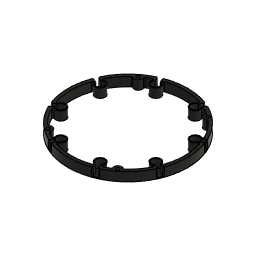
IR隠し (Autodesk Fusion 360 design; units mm, degrees)
Autodesk Fusion 360 part; units mm, degrees
sketch "スケッチ1" plane through (0, 0, 0) normal (0, 0, 1) x (1, 0, 0)
  circle A0 centre (0, 0) radius 60
  dimension "d1" = 120
  constraint coincident A0.centre origin
  measures "d1" diameter of A0
extrude "押し出し1" add sketch "スケッチ1" along normal blind 1.6 contours A0 picked at (15.326198, 22.479404)
sketch "スケッチ2" plane through (0, 0, 21.011891) normal (0, 0, 1) x (1, 0, 0)
  circle A0 centre (0, -1.188109) radius 1.5
  circle A1 centre (-35, -39.898109) radius 1.75
  circle A2 centre (35, -39.898109) radius 1.75
  circle A3 centre (-35, 45.311891) radius 1.75
  circle A4 centre (-35, -45.188109) radius 1.75
  circle A5 centre (35, 45.311891) radius 1.75
  circle A6 centre (35, -45.188109) radius 1.75
  line L0 (-40, 48.811891) -> (-40, -51.188109)
  line L1 (-40, -51.188109) -> (40, -51.188109)
  line L2 (40, -51.188109) -> (40, 48.811891)
  line L3 (40, 48.811891) -> (-40, 48.811891)
extrude "押し出し2" cut sketch "スケッチ2" against normal blind 45 contours A3 | A4 | A5 | A6 picked at (-35.557417, 45.483832) picked at (-35.557417, -45.016168) picked at (34.442583, 45.483832) picked at (34.442583, -45.016168)
sketch "スケッチ3" plane through (0, 0, 1.6) normal (0, 0, 1) x (-1, 0, 0)
  circle A0 centre (-35, 45.188109) radius 1.75
  circle A1 centre (-35, -45.311891) radius 1.75
  circle A2 centre (35, 45.188109) radius 1.75
  circle A3 centre (35, -45.311891) radius 1.75
  circle A4 centre (0, 0) radius 60
extrude "押し出し3" add sketch "スケッチ3" along normal blind 10 contours A4 picked at (11.241029, -14.670055)
extrude "押し出し4" cut 1 faces at (-11.241029, 14.670055, 11.6) along direction (0, 0, -1) blind 1.6
sketch "スケッチ4" plane through (0, 0, 10) normal (0, 0, 1) x (-1, 0, 0)
  circle A0 centre (-35, 45.188109) radius 1.75
  circle A1 centre (35, 45.188109) radius 1.75
  circle A2 centre (-35, -45.311891) radius 1.75
  circle A3 centre (35, -45.311891) radius 1.75
  circle A4 centre (0, 0) radius 60
  circle A5 centre (0, 0) radius 50
  dimension "d10" = 100
  constraint concentric A4 A5
  measures "d10" diameter of A5
extrude "押し出し5" cut sketch "スケッチ4" against normal blind 55 contours A5 picked at (-13.551782, -2.484038)
extrude "押し出し6" cut 1 faces at (-56.443283, 2.980845, 10) along direction (0, 0, -1) blind 1
sketch "スケッチ5" plane through (0, 0, 9) normal (0, 0, 1) x (-1, 0, 0)
  circle A0 centre (0, 0) radius 50
  circle A1 centre (-35, 45.188109) radius 1.75
  circle A2 centre (35, 45.188109) radius 1.75
  circle A3 centre (-35, -45.311891) radius 1.75
  circle A4 centre (35, -45.311891) radius 1.75
  circle A5 centre (0, 0) radius 60
  line L0 (0, 0) -> (0, 60)
  line L1 (0, 0) -> (22.961006, 55.432772)
  circle A6 centre (0, 0) radius 51.6
  circle A7 centre (19.746465, 47.672184) radius 4
  circle A8 centre (19.746465, 47.672184) radius 5
  circle A9 centre (-19.746465, 47.672184) radius 4
  circle A10 centre (-19.746465, 47.672184) radius 5
  circle A11 centre (-47.672184, 19.746465) radius 4
  circle A12 centre (-47.672184, 19.746465) radius 5
  circle A13 centre (-47.672184, -19.746465) radius 4
  circle A14 centre (-47.672184, -19.746465) radius 5
  circle A15 centre (-19.746465, -47.672184) radius 4
  circle A16 centre (-19.746465, -47.672184) radius 5
  circle A17 centre (19.746465, -47.672184) radius 4
  circle A18 centre (19.746465, -47.672184) radius 5
  circle A19 centre (47.672184, -19.746465) radius 4
  circle A20 centre (47.672184, -19.746465) radius 5
  circle A21 centre (47.672184, 19.746465) radius 4
  circle A22 centre (47.672184, 19.746465) radius 5
  dimension "d15" = 157.5
  dimension "d16" = 103.2
  dimension "d17" = 8
  dimension "d18" = 10
  dimension "d20" = 360
  constraint coincident A0.centre A5.centre
  constraint coincident A5 L0.end
  constraint vertical L0
  constraint concentric A7 A8
  measures "d15" angle of L0 L1
  measures "d16" diameter of A6
  measures "d17" diameter of A7
  measures "d18" diameter of A8
extrude "押し出し7" add sketch "スケッチ5" against normal blind 9 contours A0 A21 A22 | A0 A19 A20 | A0 L1 A7 A8 | A0 A17 A18 | A0 L1 A7 A8 | A0 A15 A16 | A0 A9 A10 | A0 A13 A14 | A0 A11 A12 picked at (43.248058, 18.291237) picked at (43.248058, -18.291237) picked at (22.313928, 43.786523) picked at (18.291237, -43.248058) picked at (15.183418, 46.740077) picked at (-22.308999, -43.783035) picked at (-22.308999, 43.783035) picked at (-46.768608, -15.177005) picked at (-46.768608, 15.177005)
extrude "押し出し8" cut sketch "スケッチ5" against normal blind 21 contours A0 A6 A21 | A0 A6 A19 | A6 A21 | A6 A19 | A0 L1 A6 A7 | A0 A6 A17 | A0 L1 A6 A7 | L1 A6 A7 | A6 A17 | L1 A6 A7 | A0 A6 A15 | A6 A15 | A0 A6 A9 | A6 A9 | A6 A13 | A0 A6 A13 | A0 A6 A11 | A6 A11 picked at (45.983245, 21.335973) picked at (45.983245, -21.335973) picked at (48.874047, 20.296753) picked at (48.874047, -20.296753) picked at (22.104519, 45.630587) picked at (17.428253, -47.601875) picked at (16.635442, 47.895953) picked at (21.000795, 48.527452) picked at (20.25766, -48.89118) picked at (19.466775, 49.163647) picked at (-21.335973, -45.983245) picked at (-20.252313, -48.893408) picked at (-21.335973, 45.983245) picked at (-20.252313, 48.893408) picked at (-48.893408, -20.252313) picked at (-47.601875, -17.428253) picked at (-47.601875, 17.428253) picked at (-48.893408, 20.252313)
sketch "スケッチ6" plane through (0, 0, 9) normal (0, 0, 1) x (-1, 0, 0)
  circle A0 centre (19.746465, -47.672184) radius 4
  circle A1 centre (19.746465, 47.672184) radius 4
  circle A2 centre (-47.672184, 19.746465) radius 4
  circle A3 centre (47.672184, -19.746465) radius 4
  circle A4 centre (-19.746465, -47.672184) radius 4
  circle A5 centre (-19.746465, 47.672184) radius 4
  circle A6 centre (-47.672184, -19.746465) radius 4
  circle A7 centre (47.672184, 19.746465) radius 4
  arc A8 (-23.354385, 44.21055) -> (-44.21055, 23.354385) centre (0, 0) ccw
  arc A9 (-23.354385, 44.21055) -> (-14.747535, 47.775624) centre (-19.746465, 47.672184) ccw
  arc A10 (14.747535, 47.775624) -> (-14.747535, 47.775624) centre (0, 0) ccw
  arc A11 (14.747535, 47.775624) -> (23.354385, 44.21055) centre (19.746465, 47.672184) ccw
  arc A12 (44.21055, 23.354385) -> (23.354385, 44.21055) centre (0, 0) ccw
  arc A13 (44.21055, 23.354385) -> (47.775624, 14.747535) centre (47.672184, 19.746465) ccw
  arc A14 (47.775624, -14.747535) -> (47.775624, 14.747535) centre (0, 0) ccw
  arc A15 (47.775624, -14.747535) -> (44.21055, -23.354385) centre (47.672184, -19.746465) ccw
  arc A16 (23.354385, -44.21055) -> (44.21055, -23.354385) centre (0, 0) ccw
  arc A17 (23.354385, -44.21055) -> (14.747535, -47.775624) centre (19.746465, -47.672184) ccw
  arc A18 (-14.747535, -47.775624) -> (14.747535, -47.775624) centre (0, 0) ccw
  arc A19 (-14.747535, -47.775624) -> (-23.354385, -44.21055) centre (-19.746465, -47.672184) ccw
  arc A20 (-44.21055, -23.354385) -> (-23.354385, -44.21055) centre (0, 0) ccw
  arc A21 (-44.21055, -23.354385) -> (-47.775624, -14.747535) centre (-47.672184, -19.746465) ccw
  arc A22 (-47.775624, 14.747535) -> (-47.775624, -14.747535) centre (0, 0) ccw
  arc A23 (-47.775624, 14.747535) -> (-44.21055, 23.354385) centre (-47.672184, 19.746465) ccw
  circle A24 centre (-35, 45.188109) radius 1.75
  circle A25 centre (35, 45.188109) radius 1.75
  circle A26 centre (-35, -45.311891) radius 1.75
  circle A27 centre (35, -45.311891) radius 1.75
  circle A28 centre (0, 0) radius 60
  line L0 (0, 0) -> (19.746465, 47.672184)
  line L1 (19.746465, 47.672184) -> (30.643995, 73.981148)
  line L2 (22.961006, 55.432772) -> (21.277199, 51.367702)
  line L3 (22.119102, 53.400237) -> (23.966861, 52.63487)
  line L4 (22.119102, 53.400237) -> (20.271343, 54.165604)
  line L5 (20.271343, 54.165604) -> (21.100487, 56.167334)
  line L6 (23.966861, 52.63487) -> (24.796005, 54.636601)
  line L7 (23.966861, 52.63487) -> (22.919878, 50.10723)
  line L8 (20.271343, 54.165604) -> (19.22436, 51.637963)
  line L9 (-23.966861, 52.63487) -> (-24.796005, 54.636601)
  line L10 (-23.966861, 52.63487) -> (-22.919878, 50.10723)
  line L11 (-20.271343, 54.165604) -> (-21.100487, 56.167334)
  line L12 (-20.271343, 54.165604) -> (-19.22436, 51.637963)
  line L13 (-54.165604, 20.271343) -> (-56.167334, 21.100487)
  line L14 (-54.165604, 20.271343) -> (-51.637963, 19.22436)
  line L15 (-52.63487, 23.966861) -> (-54.636601, 24.796005)
  line L16 (-52.63487, 23.966861) -> (-50.10723, 22.919878)
  line L17 (-52.63487, -23.966861) -> (-54.636601, -24.796005)
  line L18 (-52.63487, -23.966861) -> (-50.10723, -22.919878)
  line L19 (-54.165604, -20.271343) -> (-56.167334, -21.100487)
  line L20 (-54.165604, -20.271343) -> (-51.637963, -19.22436)
  line L21 (-20.271343, -54.165604) -> (-21.100487, -56.167334)
  line L22 (-20.271343, -54.165604) -> (-19.22436, -51.637963)
  line L23 (-23.966861, -52.63487) -> (-24.796005, -54.636601)
  line L24 (-23.966861, -52.63487) -> (-22.919878, -50.10723)
  line L25 (23.966861, -52.63487) -> (24.796005, -54.636601)
  line L26 (23.966861, -52.63487) -> (22.919878, -50.10723)
  line L27 (20.271343, -54.165604) -> (21.100487, -56.167334)
  line L28 (20.271343, -54.165604) -> (19.22436, -51.637963)
  line L29 (54.165604, -20.271343) -> (56.167334, -21.100487)
  line L30 (54.165604, -20.271343) -> (51.637963, -19.22436)
  line L31 (52.63487, -23.966861) -> (54.636601, -24.796005)
  line L32 (52.63487, -23.966861) -> (50.10723, -22.919878)
  line L33 (52.63487, 23.966861) -> (54.636601, 24.796005)
  line L34 (52.63487, 23.966861) -> (50.10723, 22.919878)
  line L35 (54.165604, 20.271343) -> (56.167334, 21.100487)
  line L36 (54.165604, 20.271343) -> (51.637963, 19.22436)
  dimension "d25" = 2
  dimension "d26" = 2
  dimension "d28" = 360
  constraint coincident A8.centre A10.centre
  constraint parallel L0 L1
  constraint perpendicular L1 L3
  constraint perpendicular L1 L4
  constraint perpendicular L4 L5
  constraint perpendicular L3 L6
  constraint perpendicular L3 L7
  constraint perpendicular L4 L8
extrude "押し出し9" cut sketch "スケッチ6" against normal blind 8 contours A0 A28 L25 L26 L27 L28 | A4 A28 L21 L22 L23 L24 | A3 A28 L29 L30 L31 L32 | A6 A28 L17 L18 L19 L20 | A7 A28 L33 L34 L35 L36 | A2 A28 L13 L14 L15 L16 | A28 L1 L2 L3 L6 | A5 A28 L9 L10 L11 L12 | A28 L1 L2 L4 L5 | A1 L1 L2 L3 L7 | A1 L1 L2 L4 L8 picked at (21.744986, -52.757411) picked at (-21.744986, -52.757411) picked at (52.722725, -21.838468) picked at (-52.68115, -21.929097) picked at (52.722725, 21.838468) picked at (-52.757411, 21.744986) picked at (23.424422, 53.647963) picked at (-21.929097, 52.68115) picked at (21.371271, 54.498406) picked at (22.61081, 52.390464) picked at (21.057396, 53.033909)
sketch "スケッチ7" plane through (0, 0, 0) normal (0, 0, -1) x (1, 0, 0)
  circle A0 centre (47.672184, 19.746465) radius 4
  circle A1 centre (-47.672184, -19.746465) radius 4
  circle A2 centre (19.746465, 47.672184) radius 4
  circle A3 centre (-19.746465, -47.672184) radius 4
  circle A4 centre (47.672184, -19.746465) radius 4
  circle A5 centre (-47.672184, 19.746465) radius 4
  circle A6 centre (-19.746465, 47.672184) radius 4
  circle A7 centre (19.746465, -47.672184) radius 4
  arc A8 (44.21055, 23.354385) -> (47.775624, 14.747535) centre (47.672184, 19.746465) ccw
  arc A9 (47.775624, -14.747535) -> (47.775624, 14.747535) centre (0, 0) ccw
  arc A10 (47.775624, -14.747535) -> (44.21055, -23.354385) centre (47.672184, -19.746465) ccw
  arc A11 (23.354385, -44.21055) -> (44.21055, -23.354385) centre (0, 0) ccw
  arc A12 (23.354385, -44.21055) -> (14.747535, -47.775624) centre (19.746465, -47.672184) ccw
  arc A13 (-14.747535, -47.775624) -> (14.747535, -47.775624) centre (0, 0) ccw
  arc A14 (-14.747535, -47.775624) -> (-23.354385, -44.21055) centre (-19.746465, -47.672184) ccw
  arc A15 (-44.21055, -23.354385) -> (-23.354385, -44.21055) centre (0, 0) ccw
  arc A16 (-44.21055, -23.354385) -> (-47.775624, -14.747535) centre (-47.672184, -19.746465) ccw
  arc A17 (-47.775624, 14.747535) -> (-47.775624, -14.747535) centre (0, 0) ccw
  arc A18 (-47.775624, 14.747535) -> (-44.21055, 23.354385) centre (-47.672184, 19.746465) ccw
  arc A19 (-23.354385, 44.21055) -> (-44.21055, 23.354385) centre (0, 0) ccw
  arc A20 (-23.354385, 44.21055) -> (-14.747535, 47.775624) centre (-19.746465, 47.672184) ccw
  arc A21 (14.747535, 47.775624) -> (-14.747535, 47.775624) centre (0, 0) ccw
  arc A22 (14.747535, 47.775624) -> (23.354385, 44.21055) centre (19.746465, 47.672184) ccw
  arc A23 (44.21055, 23.354385) -> (23.354385, 44.21055) centre (0, 0) ccw
  circle A24 centre (35, 45.188109) radius 1.75
  circle A25 centre (35, -45.311891) radius 1.75
  circle A26 centre (-35, 45.188109) radius 1.75
  circle A27 centre (-35, -45.311891) radius 1.75
  circle A28 centre (0, 0) radius 60
extrude "押し出し10" add sketch "スケッチ7" against normal blind 1 contours A0 | A1 | A2 | A3 | A4 | A5 | A6 | A7 picked at (48.338851, 21.687179) picked at (-48.901937, -19.945188) picked at (18.600469, 46.726807) picked at (-18.915145, -49.112072) picked at (46.442431, -19.945188) picked at (-47.005517, 21.687179) picked at (-18.915145, 46.232296) picked at (18.545173, -47.853249)
sketch "スケッチ8" plane through (0, 0, 9) normal (0, 0, 1) x (-1, 0, 0)
  circle A0 centre (35, -45.311891) radius 1.75
  circle A1 centre (-35, -45.311891) radius 1.75
  circle A2 centre (35, 45.188109) radius 1.75
  circle A3 centre (-35, 45.188109) radius 1.75
  arc A4 (-23.354385, 44.21055) -> (-44.21055, 23.354385) centre (0, 0) ccw
  arc A5 (-23.354385, 44.21055) -> (-14.747535, 47.775624) centre (-19.746465, 47.672184) ccw
  arc A6 (14.747535, 47.775624) -> (-14.747535, 47.775624) centre (0, 0) ccw
  arc A7 (14.747535, 47.775624) -> (23.354385, 44.21055) centre (19.746465, 47.672184) ccw
  arc A8 (44.21055, 23.354385) -> (23.354385, 44.21055) centre (0, 0) ccw
  arc A9 (44.21055, 23.354385) -> (47.775624, 14.747535) centre (47.672184, 19.746465) ccw
  arc A10 (47.775624, -14.747535) -> (47.775624, 14.747535) centre (0, 0) ccw
  arc A11 (47.775624, -14.747535) -> (44.21055, -23.354385) centre (47.672184, -19.746465) ccw
  arc A12 (23.354385, -44.21055) -> (44.21055, -23.354385) centre (0, 0) ccw
  arc A13 (23.354385, -44.21055) -> (14.747535, -47.775624) centre (19.746465, -47.672184) ccw
  arc A14 (-14.747535, -47.775624) -> (14.747535, -47.775624) centre (0, 0) ccw
  arc A15 (-14.747535, -47.775624) -> (-23.354385, -44.21055) centre (-19.746465, -47.672184) ccw
  arc A16 (-44.21055, -23.354385) -> (-23.354385, -44.21055) centre (0, 0) ccw
  arc A17 (-44.21055, -23.354385) -> (-47.775624, -14.747535) centre (-47.672184, -19.746465) ccw
  arc A18 (-47.775624, 14.747535) -> (-47.775624, -14.747535) centre (0, 0) ccw
  arc A19 (-47.775624, 14.747535) -> (-44.21055, 23.354385) centre (-47.672184, 19.746465) ccw
  line L0 (-56.167334, -21.100487) -> (-51.637963, -19.22436)
  arc A20 (-50.10723, -22.919878) -> (-51.637963, -19.22436) centre (-47.672184, -19.746465) ccw
  line L1 (-50.10723, -22.919878) -> (-54.636601, -24.796005)
  arc A21 (-54.636601, -24.796005) -> (-24.796005, -54.636601) centre (0, 0) ccw
  line L2 (-24.796005, -54.636601) -> (-22.919878, -50.10723)
  arc A22 (-19.22436, -51.637963) -> (-22.919878, -50.10723) centre (-19.746465, -47.672184) ccw
  line L3 (-19.22436, -51.637963) -> (-21.100487, -56.167334)
  arc A23 (-21.100487, -56.167334) -> (21.100487, -56.167334) centre (0, 0) ccw
  line L4 (21.100487, -56.167334) -> (19.22436, -51.637963)
  arc A24 (22.919878, -50.10723) -> (19.22436, -51.637963) centre (19.746465, -47.672184) ccw
  line L5 (22.919878, -50.10723) -> (24.796005, -54.636601)
  arc A25 (24.796005, -54.636601) -> (54.636601, -24.796005) centre (0, 0) ccw
  line L6 (54.636601, -24.796005) -> (50.10723, -22.919878)
  arc A26 (51.637963, -19.22436) -> (50.10723, -22.919878) centre (47.672184, -19.746465) ccw
  line L7 (51.637963, -19.22436) -> (56.167334, -21.100487)
  arc A27 (56.167334, -21.100487) -> (56.167334, 21.100487) centre (0, 0) ccw
  line L8 (56.167334, 21.100487) -> (51.637963, 19.22436)
  arc A28 (50.10723, 22.919878) -> (51.637963, 19.22436) centre (47.672184, 19.746465) ccw
  line L9 (50.10723, 22.919878) -> (54.636601, 24.796005)
  arc A29 (54.636601, 24.796005) -> (24.796005, 54.636601) centre (0, 0) ccw
  line L10 (24.796005, 54.636601) -> (22.919878, 50.10723)
  arc A30 (19.22436, 51.637963) -> (22.919878, 50.10723) centre (19.746465, 47.672184) ccw
  line L11 (19.22436, 51.637963) -> (21.100487, 56.167334)
  arc A31 (21.100487, 56.167334) -> (-21.100487, 56.167334) centre (0, 0) ccw
  line L12 (-21.100487, 56.167334) -> (-19.22436, 51.637963)
  arc A32 (-22.919878, 50.10723) -> (-19.22436, 51.637963) centre (-19.746465, 47.672184) ccw
  line L13 (-22.919878, 50.10723) -> (-24.796005, 54.636601)
  arc A33 (-24.796005, 54.636601) -> (-54.636601, 24.796005) centre (0, 0) ccw
  line L14 (-54.636601, 24.796005) -> (-50.10723, 22.919878)
  arc A34 (-51.637963, 19.22436) -> (-50.10723, 22.919878) centre (-47.672184, 19.746465) ccw
  line L15 (-51.637963, 19.22436) -> (-56.167334, 21.100487)
  arc A35 (-56.167334, 21.100487) -> (-56.167334, -21.100487) centre (0, 0) ccw
  circle A36 centre (0, 0) radius 60
  circle A37 centre (0, 0) radius 57
  circle A38 centre (-19.746465, 47.672184) radius 5
  circle A39 centre (19.746465, 47.672184) radius 5
  circle A40 centre (47.672184, 19.746465) radius 5
  circle A41 centre (47.672184, -19.746465) radius 5
  circle A42 centre (19.746465, -47.672184) radius 5
  circle A43 centre (-19.746465, -47.672184) radius 5
  circle A44 centre (-47.672184, -19.746465) radius 5
  circle A45 centre (-47.672184, 19.746465) radius 5
  circle A46 centre (35, 45.188109) radius 4
  circle A47 centre (-35, 45.188109) radius 4
  circle A48 centre (-35, -45.311891) radius 4
  circle A49 centre (35, -45.311891) radius 4
  line L16 (19.746465, 47.672184) -> (16.974827, 48.820234)
  line L17 (19.746465, 47.672184) -> (22.518104, 46.524134)
  line L18 (22.518104, 46.524134) -> (24.554361, 51.440095)
  line L19 (16.974827, 48.820234) -> (19.011084, 53.736195)
  line L20 (-22.518104, 46.524134) -> (-24.554361, 51.440095)
  line L21 (-16.974827, 48.820234) -> (-19.011084, 53.736195)
  line L22 (-48.820234, 16.974827) -> (-53.736195, 19.011084)
  line L23 (-46.524134, 22.518104) -> (-51.440095, 24.554361)
  line L24 (-46.524134, -22.518104) -> (-51.440095, -24.554361)
  line L25 (-48.820234, -16.974827) -> (-53.736195, -19.011084)
  line L26 (-16.974827, -48.820234) -> (-19.011084, -53.736195)
  line L27 (-22.518104, -46.524134) -> (-24.554361, -51.440095)
  line L28 (22.518104, -46.524134) -> (24.554361, -51.440095)
  line L29 (16.974827, -48.820234) -> (19.011084, -53.736195)
  line L30 (48.820234, -16.974827) -> (53.736195, -19.011084)
  line L31 (46.524134, -22.518104) -> (51.440095, -24.554361)
  line L32 (46.524134, 22.518104) -> (51.440095, 24.554361)
  line L33 (48.820234, 16.974827) -> (53.736195, 19.011084)
  dimension "d33" = 114
  dimension "d34" = 8
  dimension "d35" = 8
  dimension "d36" = 8
  dimension "d37" = 8
  dimension "d38" = 3
  dimension "d39" = 3
  dimension "d41" = 360
  constraint concentric A4 A36
  constraint concentric A4 A37
  constraint concentric A5 A38
  constraint concentric A7 A39
  constraint concentric A9 A40
  constraint concentric A11 A41
  constraint concentric A13 A42
  constraint concentric A15 A43
  constraint concentric A17 A44
  constraint concentric A19 A45
  constraint concentric A2 A46
  constraint concentric A3 A47
  constraint concentric A1 A48
  constraint concentric A0 A49
  constraint perpendicular L11 L16
  constraint perpendicular L11 L17
  constraint perpendicular L17 L18
  constraint perpendicular L16 L19
  measures "d33" diameter of A37
  measures "d34" diameter of A46
  measures "d35" diameter of A47
  measures "d36" diameter of A48
  measures "d37" diameter of A49
extrude "押し出し11" cut sketch "スケッチ8" against normal blind 20 contours A12 A37 A41 A42 A49 L28 L31 | A10 A37 A40 A41 L30 L33 | A14 A37 A42 A43 L26 L29 | A8 A37 A39 A40 A46 L18 L32 | A16 A37 A43 A44 A48 L24 L27 | A6 A37 A38 A39 L19 L21 | A4 A37 A38 A45 A47 L20 L23 | A18 A37 A44 A45 L22 L25 picked at (39.597657, -34.074082) picked at (52.025004, -4.634722) picked at (0, -54.578822) picked at (39.609815, 34.05994) picked at (-39.597657, -34.074082) picked at (0, 54.578822) picked at (-39.609815, 34.05994) picked at (-54.578822, 0)
fillet "フィレット1" radius 1 40 edges at (-24.554361, -51.440095, 4.5) (-24.048837, -50.219652, 4.5) (-19.011084, -53.736195, 4.5) (-18.50556, -52.515752, 4.5) (-31.664432, -47.39582, 4.5) (-37.971688, -42.510597, 4.5) (-53.736195, -19.011084, 4.5) (-52.515752, -18.50556, 4.5) (-51.440095, -24.554361, 4.5) (-50.219652, -24.048837, 4.5) (-53.736195, 19.011084, 4.5) (-52.515752, 18.50556, 4.5) (-51.440095, 24.554361, 4.5) (-50.219652, 24.048837, 4.5) (-31.608705, 47.433003, 4.5) (-19.011084, 53.736195, 4.5) (-18.50556, 52.515752, 4.5) (-37.909056, 42.56646, 4.5) (-24.554361, 51.440095, 4.5) (-24.048837, 50.219652, 4.5) (19.011084, 53.736195, 4.5) (18.50556, 52.515752, 4.5) (31.608705, 47.433003, 4.5) (24.554361, 51.440095, 4.5) (24.048837, 50.219652, 4.5) (37.909056, 42.56646, 4.5) (52.515752, 18.50556, 4.5) (53.736195, 19.011084, 4.5) (51.440095, 24.554361, 4.5) (50.219652, 24.048837, 4.5) (53.736195, -19.011084, 4.5) (52.515752, -18.50556, 4.5) (51.440095, -24.554361, 4.5) (50.219652, -24.048837, 4.5) (31.664432, -47.39582, 4.5) (37.971688, -42.510597, 4.5) (19.011084, -53.736195, 4.5) (18.50556, -52.515752, 4.5) (24.554361, -51.440095, 4.5) (24.048837, -50.219652, 4.5)
fillet "フィレット2" radius 1 4 edges at (-22.919878, -50.10723, 5) (-24.796005, -54.636601, 5) (-21.100487, -56.167334, 5) (-19.22436, -51.637963, 5)
sketch "スケッチ9" plane through (0, 0, 9) normal (0, 0, 1) x (-1, 0, 0)
  arc A0 (-24.36761, 49.581377) -> (-17.828825, 52.28983) centre (-19.746465, 47.672184) ccw
  arc A1 (-17.75682, 54.163598) -> (-17.828825, 52.28983) centre (-17.445297, 53.213359) ccw
  arc A2 (17.75682, 54.163598) -> (-17.75682, 54.163598) centre (0, 0) ccw
  arc A3 (17.828825, 52.28983) -> (17.75682, 54.163598) centre (17.445297, 53.213359) ccw
  arc A4 (17.828825, 52.28983) -> (24.36761, 49.581377) centre (19.746465, 47.672184) ccw
  arc A5 (25.743479, 50.855415) -> (24.36761, 49.581377) centre (25.291839, 49.963215) ccw
  arc A6 (30.903775, 47.895268) -> (25.743479, 50.855415) centre (0, 0) ccw
  arc A7 (31.289283, 46.681622) -> (30.903775, 47.895268) centre (30.361604, 47.055) ccw
  arc A8 (31.289283, 46.681622) -> (37.373995, 41.968769) centre (35, 45.188109) ccw
  arc A9 (38.645484, 41.899004) -> (37.373995, 41.968769) centre (37.967493, 41.163934) ccw
  arc A10 (50.855415, 25.743479) -> (38.645484, 41.899004) centre (0, 0) ccw
  arc A11 (49.581377, 24.36761) -> (50.855415, 25.743479) centre (49.963215, 25.291839) ccw
  arc A12 (49.581377, 24.36761) -> (52.28983, 17.828825) centre (47.672184, 19.746465) ccw
  arc A13 (54.163598, 17.75682) -> (52.28983, 17.828825) centre (53.213359, 17.445297) ccw
  arc A14 (54.163598, -17.75682) -> (54.163598, 17.75682) centre (0, 0) ccw
  arc A15 (52.28983, -17.828825) -> (54.163598, -17.75682) centre (53.213359, -17.445297) ccw
  arc A16 (52.28983, -17.828825) -> (49.581377, -24.36761) centre (47.672184, -19.746465) ccw
  arc A17 (50.855415, -25.743479) -> (49.581377, -24.36761) centre (49.963215, -25.291839) ccw
  arc A18 (38.568838, -41.969569) -> (50.855415, -25.743479) centre (0, 0) ccw
  arc A19 (37.313753, -42.048987) -> (38.568838, -41.969569) centre (37.892192, -41.233261) ccw
  arc A20 (37.313753, -42.048987) -> (31.258409, -46.726281) centre (35, -45.311891) ccw
  arc A21 (30.864494, -47.920591) -> (31.258409, -46.726281) centre (30.323012, -47.079879) ccw
  arc A22 (25.743479, -50.855415) -> (30.864494, -47.920591) centre (0, 0) ccw
  arc A23 (24.36761, -49.581377) -> (25.743479, -50.855415) centre (25.291839, -49.963215) ccw
  arc A24 (24.36761, -49.581377) -> (17.828825, -52.28983) centre (19.746465, -47.672184) ccw
  arc A25 (17.75682, -54.163598) -> (17.828825, -52.28983) centre (17.445297, -53.213359) ccw
  arc A26 (-17.75682, -54.163598) -> (17.75682, -54.163598) centre (0, 0) ccw
  arc A27 (-17.828825, -52.28983) -> (-17.75682, -54.163598) centre (-17.445297, -53.213359) ccw
  arc A28 (-17.828825, -52.28983) -> (-24.36761, -49.581377) centre (-19.746465, -47.672184) ccw
  arc A29 (-25.743479, -50.855415) -> (-24.36761, -49.581377) centre (-25.291839, -49.963215) ccw
  arc A30 (-30.864494, -47.920591) -> (-25.743479, -50.855415) centre (0, 0) ccw
  arc A31 (-31.258409, -46.726281) -> (-30.864494, -47.920591) centre (-30.323012, -47.079879) ccw
  arc A32 (-31.258409, -46.726281) -> (-37.313753, -42.048987) centre (-35, -45.311891) ccw
  arc A33 (-38.568838, -41.969569) -> (-37.313753, -42.048987) centre (-37.892192, -41.233261) ccw
  arc A34 (-50.855415, -25.743479) -> (-38.568838, -41.969569) centre (0, 0) ccw
  arc A35 (-49.581377, -24.36761) -> (-50.855415, -25.743479) centre (-49.963215, -25.291839) ccw
  arc A36 (-49.581377, -24.36761) -> (-52.28983, -17.828825) centre (-47.672184, -19.746465) ccw
  arc A37 (-54.163598, -17.75682) -> (-52.28983, -17.828825) centre (-53.213359, -17.445297) ccw
  arc A38 (-54.163598, 17.75682) -> (-54.163598, -17.75682) centre (0, 0) ccw
  arc A39 (-52.28983, 17.828825) -> (-54.163598, 17.75682) centre (-53.213359, 17.445297) ccw
  arc A40 (-52.28983, 17.828825) -> (-49.581377, 24.36761) centre (-47.672184, 19.746465) ccw
  arc A41 (-50.855415, 25.743479) -> (-49.581377, 24.36761) centre (-49.963215, 25.291839) ccw
  arc A42 (-38.645484, 41.899004) -> (-50.855415, 25.743479) centre (0, 0) ccw
  arc A43 (-37.373995, 41.968769) -> (-38.645484, 41.899004) centre (-37.967493, 41.163934) ccw
  arc A44 (-37.373995, 41.968769) -> (-31.289283, 46.681622) centre (-35, 45.188109) ccw
  arc A45 (-30.903775, 47.895268) -> (-31.289283, 46.681622) centre (-30.361604, 47.055) ccw
  arc A46 (-25.743479, 50.855415) -> (-30.903775, 47.895268) centre (0, 0) ccw
  arc A47 (-24.36761, 49.581377) -> (-25.743479, 50.855415) centre (-25.291839, 49.963215) ccw
  arc A48 (18.753741, 51.547039) -> (19.42944, 52.133069) centre (18.50556, 52.515752) ccw
  line L0 (19.42944, 52.133069) -> (20.701357, 55.203748)
  arc A49 (20.701357, 55.203748) -> (20.112689, 56.528575) centre (19.777477, 55.586432) ccw
  arc A50 (20.112689, 56.528575) -> (-21.100487, 56.167334) centre (0, 0) ccw
  line L1 (-21.100487, 56.167334) -> (-19.22436, 51.637963)
  arc A51 (-22.919878, 50.10723) -> (-19.22436, 51.637963) centre (-19.746465, 47.672184) ccw
  line L2 (-22.919878, 50.10723) -> (-24.796005, 54.636601)
  arc A52 (-24.796005, 54.636601) -> (-54.636601, 24.796005) centre (0, 0) ccw
  line L3 (-54.636601, 24.796005) -> (-50.10723, 22.919878)
  arc A53 (-51.637963, 19.22436) -> (-50.10723, 22.919878) centre (-47.672184, 19.746465) ccw
  line L4 (-51.637963, 19.22436) -> (-56.167334, 21.100487)
  arc A54 (-56.167334, 21.100487) -> (-56.167334, -21.100487) centre (0, 0) ccw
  line L5 (-56.167334, -21.100487) -> (-51.637963, -19.22436)
  arc A55 (-50.10723, -22.919878) -> (-51.637963, -19.22436) centre (-47.672184, -19.746465) ccw
  line L6 (-50.10723, -22.919878) -> (-54.636601, -24.796005)
  arc A56 (-54.636601, -24.796005) -> (-24.796005, -54.636601) centre (0, 0) ccw
  line L7 (-24.796005, -54.636601) -> (-22.919878, -50.10723)
  arc A57 (-19.22436, -51.637963) -> (-22.919878, -50.10723) centre (-19.746465, -47.672184) ccw
  line L8 (-19.22436, -51.637963) -> (-21.100487, -56.167334)
  arc A58 (-21.100487, -56.167334) -> (21.100487, -56.167334) centre (0, 0) ccw
  line L9 (21.100487, -56.167334) -> (19.22436, -51.637963)
  arc A59 (22.919878, -50.10723) -> (19.22436, -51.637963) centre (19.746465, -47.672184) ccw
  line L10 (22.919878, -50.10723) -> (24.796005, -54.636601)
  arc A60 (24.796005, -54.636601) -> (54.636601, -24.796005) centre (0, 0) ccw
  line L11 (54.636601, -24.796005) -> (50.10723, -22.919878)
  arc A61 (51.637963, -19.22436) -> (50.10723, -22.919878) centre (47.672184, -19.746465) ccw
  line L12 (51.637963, -19.22436) -> (56.167334, -21.100487)
  arc A62 (56.167334, -21.100487) -> (56.167334, 21.100487) centre (0, 0) ccw
  line L13 (56.167334, 21.100487) -> (51.637963, 19.22436)
  arc A63 (50.10723, 22.919878) -> (51.637963, 19.22436) centre (47.672184, 19.746465) ccw
  line L14 (50.10723, 22.919878) -> (54.636601, 24.796005)
  arc A64 (54.636601, 24.796005) -> (25.74992, 54.193557) centre (0, 0) ccw
  arc A65 (25.74992, 54.193557) -> (24.396875, 53.673015) centre (25.320754, 53.290331) ccw
  line L15 (24.396875, 53.673015) -> (23.124958, 50.602335)
  arc A66 (23.124958, 50.602335) -> (23.188363, 49.710158) centre (24.048837, 50.219652) ccw
  arc A67 (18.753741, 51.547039) -> (23.188363, 49.710158) centre (19.746465, 47.672184) ccw
  circle A68 centre (-35, 45.188109) radius 1.75
  circle A69 centre (35, 45.188109) radius 1.75
  circle A70 centre (-35, -45.311891) radius 1.75
  circle A71 centre (35, -45.311891) radius 1.75
  arc A72 (-20.112689, 56.528575) -> (-20.701357, 55.203748) centre (-19.777477, 55.586432) ccw
  arc A73 (-24.396875, 53.673015) -> (-25.74992, 54.193557) centre (-25.320754, 53.290331) ccw
  arc A74 (-54.193557, 25.74992) -> (-53.673015, 24.396875) centre (-53.290331, 25.320754) ccw
  arc A75 (-55.203748, 20.701357) -> (-56.528575, 20.112689) centre (-55.586432, 19.777477) ccw
  arc A76 (-56.528575, -20.112689) -> (-55.203748, -20.701357) centre (-55.586432, -19.777477) ccw
  arc A77 (-53.673015, -24.396875) -> (-54.193557, -25.74992) centre (-53.290331, -25.320754) ccw
  arc A78 (-25.74992, -54.193557) -> (-24.396875, -53.673015) centre (-25.320754, -53.290331) ccw
  arc A79 (-20.701357, -55.203748) -> (-20.112689, -56.528575) centre (-19.777477, -55.586432) ccw
  arc A80 (20.112689, -56.528575) -> (20.701357, -55.203748) centre (19.777477, -55.586432) ccw
  arc A81 (24.396875, -53.673015) -> (25.74992, -54.193557) centre (25.320754, -53.290331) ccw
  arc A82 (54.193557, -25.74992) -> (53.673015, -24.396875) centre (53.290331, -25.320754) ccw
  arc A83 (55.203748, -20.701357) -> (56.528575, -20.112689) centre (55.586432, -19.777477) ccw
  arc A84 (56.528575, 20.112689) -> (55.203748, 20.701357) centre (55.586432, 19.777477) ccw
  arc A85 (53.673015, 24.396875) -> (54.193557, 25.74992) centre (53.290331, 25.320754) ccw
  dimension "d49" = 360
extrude "押し出し12" cut sketch "スケッチ9" against normal blind 8 contours A50 L1 A72 | L14 A64 A85 | L2 A52 A73 | A62 L13 A84 | A52 L3 A74 | L12 A62 A83 | L4 A54 A75 | A60 L11 A82 | A54 L5 A76 | L10 A60 A81 | L6 A56 A77 | A58 L9 A80 | A56 L7 A78 | L8 A58 A79 picked at (-20.843785, 56.171897) picked at (54.458311, 24.980748) picked at (-24.980748, 54.458311) picked at (56.171897, 20.843785) picked at (-54.458311, 24.980748) picked at (56.171897, -20.843785) picked at (-56.171897, 20.843785) picked at (54.458311, -24.980748) picked at (-56.171897, -20.843785) picked at (24.980748, -54.458311) picked at (-54.458311, -24.980748) picked at (20.843785, -56.171897) picked at (-24.980748, -54.458311) picked at (-20.843785, -56.171897)
